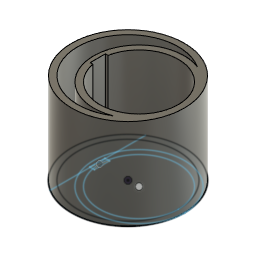
dc-15s_vibration_assembly (Autodesk Fusion 360 design; units mm, degrees)
Autodesk Fusion 360 part; units mm, degrees
sketch "Sketch1" plane through (0, 0, 0) normal (0, 1, 0) x (1, 0, 0)
  circle A0 centre (0, 0) radius 18.625
  circle A1 centre (3.6328, 0.0167) radius 13
  line L0 (-9.9984, -15.7138) -> (-9.9984, 15.7138)
  circle A2 centre (0, 0) radius 16.625
  circle A3 centre (3.6328, 0.0167) radius 15
  line L1 (-8.6172, -2.5) -> (-10.1172, -2.5)
  line L2 (-10.1172, -2.5) -> (-10.1172, 2.5)
  line L3 (-10.1172, 2.5) -> (-8.6172, 2.5)
  line L4 (-8.6172, 2.5) -> (-8.6172, -2.5)
  line L5 (-8.6172, -2.5) -> (-10.1172, 2.5) construction
  line L6 (-10.1172, -2.5) -> (-8.6172, 2.5) construction
  point P0 (-9.3672, 0)
  dimension "d1" = 37.25
  dimension "d2" = 26
  dimension "d3" = -2
  dimension "d6" = 2
  dimension "d9" = 1.5
  dimension "d10" = 5
  constraint coincident A0.centre A2.centre
  constraint coincident A0 L0.start
  constraint coincident A0 L0.end
  constraint vertical L0
  constraint horizontal L1
  constraint perpendicular L1 L2
  constraint parallel L1 L3
  constraint parallel L2 L4
  constraint coincident L5 P0
  constraint coincident L6 P0
  constraint coincident A1 P0
  measures "d1" diameter of A0
  measures "d2" diameter of A1
  measures "d9" distance of L2.end L3.end
  measures "d10" distance of L1.end L2.end
extrude "Extrude2" add sketch "Sketch1" along normal blind 2 contours A1 A2 L1 L3 L4 | A1 L0 L1 L3 | A1 L1 L3 L4
extrude "Extrude1" add sketch "Sketch1" along normal blind 30 contours A0 L0 A2 | A0 L0 A2 A3 | A0 L0 A2 A3 | A0 A1 A2 A3 | A1 L0 A2 A3 L3 | L0 A3 L1 L2 L3 | A1 L0 A2 A3 L1 | L0 L1 L2 L3
